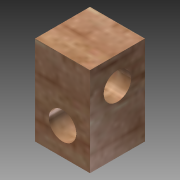
# Autodesk Inventor part: BarClamp
Saved by Autodesk Inventor 2014 (Build 180170000, 170)
## iProperties
Created: 2013-12-17
Part Number: BarClamp
Material: Birch
Document SubType Name: Modeling
Designer: Bram
Density: 0.512 g/cm^3
Appearance: Birch - Natural Medium Gloss
Author: Bram
Autodesk Inventor part; units mm, degrees
ref_plane "YZ Plane" through (0, 0, 0) normal (1, 0, 0) x (0, 1, 0)
ref_plane "XZ Plane" through (0, 0, 0) normal (0, 1, 0) x (-1, 0, 0)
ref_plane "XY Plane" through (0, 0, 0) normal (0, 0, 1) x (1, 0, 0)
sketch "Sketch1" plane through (0, 0, 0) normal (1, 0, 0) x (0, 1, 0)
  line L0 (0, 0) -> (16, 0)
  line L1 (16, 0) -> (16, 26)
  line L2 (16, 26) -> (0, 26)
  line L3 (0, 26) -> (0, 0)
  circle A0 centre (8, 18) radius 4
  dimension "d0" = 16
  dimension "d1" = 26
  dimension "d4" = 8
  constraints: 8 end point, 2 parallel, 1 centre point, 1 horizontal, 1 perpendicular
  measures "d0" distance of L2.end L1.end
  measures "d1" distance of L1.end L0.end
  measures "d4" diameter of A0
extrude "Extrusion1" add sketch "Sketch1" along normal blind 16
sketch "Sketch2" plane through (0, 16, 26) normal (0, 1, 0) x (1, 0, 0)
  circle A0 centre (8, 18) radius 4
  dimension "d8" = 8
  constraints: 1 centre point
  measures "d8" diameter of A0
extrude "Extrusion2" cut sketch "Sketch2" against normal blind 16
body "Solid1"
